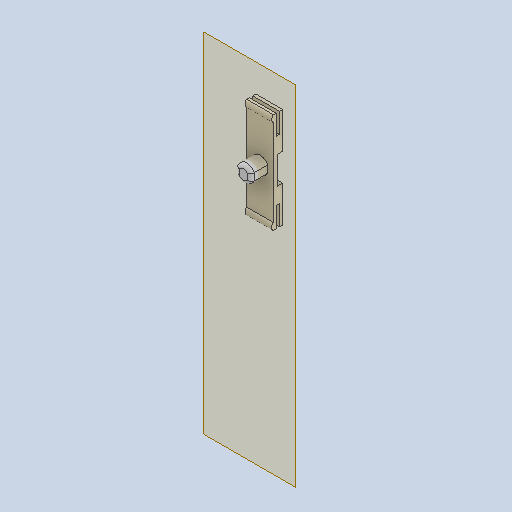
# Autodesk Inventor part: ON_Off_switch
Saved by Autodesk Inventor 2022 (Build 260153000, 153)
## iProperties
Created: 2020-11-26
Part Number: ON_Off_switch
Material: Generic
Document SubType Name: Modeling
Designer: simen
Density: 1 g/cm^3
Appearance: Default
Author: simen
## iProperties of the stored document ON_Off_switch_3DPrint.ipt
Created: 2021-12-08
Part Number: ON_Off_switch_3DPrint
Material: Generic
Document SubType Name: Modeling
Designer: simen
Density: 1 g/cm^3
Appearance: Default
Author: simen
Autodesk Inventor part; units mm, degrees
ref_plane "YZ Plane" through (0, 0, 0) normal (1, 0, 0) x (0, 1, 0)
ref_plane "XZ Plane" through (0, 0, 0) normal (0, 1, 0) x (-1, 0, 0)
ref_plane "XY Plane" through (0, 0, 0) normal (0, 0, 1) x (1, 0, 0)
ref_plane "Work Plane1" through (0, 0, 0) normal (0, 0, 1) x (1, 0, 0)
sketch "Sketch1" plane through (0, 0, 0) normal (0, 0, 1) x (1, 0, 0)
  circle A0 centre (12.6053, 80.6735) radius 2.5
  point P0 (0, 0)
  dimension "d0" = 5
  constraints: 1 centre point
  measures "d0" diameter of A0
extrude "Extrusion1" add sketch "Sketch1" along normal blind 2 and the other way blind 3
sketch "Sketch2" plane through (12.6053, 80.6735, -3) normal (0, 0, -1) x (-1, 0, 0)
  line L0 (-4, -15) -> (4, -15)
  line L1 (4, -15) -> (4, 15)
  line L2 (4, 15) -> (-4, 15)
  line L3 (-4, 15) -> (-4, -15)
  line L4 (-4, -15) -> (4, 15)
  line L5 (-4, -15) -> (27.0483, -15) construction
  circle A0 centre (0, 0) radius 2.5 projected
  point P0 (12.6053, -80.6735)
  dimension "d5" = 8
  dimension "d6" = 30
  constraints: 12 end point, 2 horizontal, 2 parallel, 1 coincident, 1 equal length, 1 midpoint, 1 perpendicular
  measures "d5" distance of L0.start L0.end
  measures "d6" distance of L0.end L1.end
extrude "Extrusion2" add sketch "Sketch2" along normal blind 2.75
sketch "Sketch5" plane through (12.6053, 80.6735, 2) normal (0, 0, 1) x (1, 0, 0)
  line L0 (4, 15) -> (4, -15) projected
  line L1 (-4, -15) -> (-4, 15) projected
  circle A0 centre (0, 0) radius 2.5 projected
  line L2 (-2.25, 1.0897) -> (-2.25, -1.0897)
  line L3 (2.25, 1.0897) -> (2.25, -1.0897)
  circle A1 centre (0, 0) radius 2.5 projected
  point P0 (-12.6053, -80.6735)
  point P1 (2.25, 1.0897)
  point P2 (2.25, -1.0897)
  point P3 (-2.25, -1.0897)
  point P4 (-2.25, 1.0897)
  dimension "d21" = 1.75
  dimension "d22" = 1.75
  constraints: 4 end point, 4 point on circle, 2 parallel, 1 vertical
  measures "d21" distance between parallel lines of L1 L2
  measures "d22" distance between parallel lines of L0 L3
extrude "Extrusion5" cut sketch "Sketch5" against normal up to surface (5 mm away) contours A0 L3 | L2 A0
fillet "Fillet1" radius 1 4 edges at (12.6053, 83.1735, 2) (12.6053, 78.1735, 2) (10.3553, 80.6735, 2) (14.8553, 80.6735, 2)
sketch "Sketch7" plane through (16.6053, 65.6735, -3) normal (1, 0, 0) x (0, 0, -1)
  line L0 (3.95, 19.8) -> (5.45, 19.8) construction
  line L1 (1.25, 19.15) -> (1.25, 10.85)
  line L2 (0, 30) -> (2.75, 30) projected
  line L3 (0, 30) -> (0, 0) projected
  line L4 (0, 0) -> (2.75, 0) projected
  line L5 (2.75, 30) -> (2.75, 0) projected
  line L6 (0, 30) -> (2.75, 30) projected
  line L7 (1.25, 19.15) -> (2.75, 19.15)
  line L8 (2.75, 30) -> (2.75, 0) projected
  line L9 (1.25, 10.85) -> (2.75, 10.85)
  point P0 (-3, -65.6735)
  point P1 (2.75, 10.85)
  point P2 (2.75, 19.15)
  dimension "d31" = 8.3
  dimension "d52" = 1.5
  dimension "d53" = 10.85
  constraints: 8 end point, 2 parallel, 2 point on line, 1 horizontal, 1 perpendicular
  measures "d31" distance of L1.start L1.end
  measures "d52" distance of L1.end L9.end
  measures "d53" distance between parallel lines of L2 L7
extrude "Extrusion7" cut sketch "Sketch7" against normal blind 5 contours L7 L5 L9 L1
chamfer "Chamfer1" distance 0.7 angle 45 1 edges at (11.6053, 80.6735, -4.25)
sketch "Sketch8" plane through (16.6053, 65.6735, -3) normal (1, 0, 0) x (0, 0, -1)
  line L0 (0, 30) -> (2.75, 30) projected
  line L1 (0, 30) -> (0, 0) projected
  line L2 (0, 0) -> (2.75, 0) projected
  line L3 (0, 0) -> (2.75, 0) projected
  line L4 (0, 30) -> (2.75, 30) projected
  line L5 (0.8, 0) -> (0.8, 30)
  line L6 (0, 30) -> (0, 0) projected
  line L7 (1.8, 0) -> (1.8, 30)
  line L8 (0.8, 6) -> (1.8, 6)
  line L9 (0.8, 24) -> (1.8, 24)
  line L10 (2.75, 30) -> (2.75, 19.15) projected
  line L11 (2.75, 10.85) -> (1.25, 10.85) projected
  line L12 (1.25, 10.85) -> (1.25, 19.15) projected
  line L13 (1.25, 19.15) -> (2.75, 19.15) projected
  line L14 (2.75, 10.85) -> (2.75, 0) projected
  point P0 (-3, -65.6735)
  dimension "d38" = 0.8
  dimension "d39" = 1
  dimension "d40" = 6
  dimension "d41" = 6
  dimension "d55" = 0.95
  constraints: 8 end point, 8 point on line, 2 parallel, 2 perpendicular
  measures "d38" distance between parallel lines of L1 L5
  measures "d39" distance between parallel lines of L5 L7
  measures "d40" distance between parallel lines of L2 L8
  measures "d41" distance between parallel lines of L0 L9
  measures "d55" distance between parallel lines of L14 L7
extrude "Extrusion8" cut sketch "Sketch8" against normal up to surface (8 mm away) contours L0 L7 L9 L5 | L5 L8 L7 L2
sketch "Sketch9" plane through (16.6053, 65.6735, -3) normal (1, 0, 0) x (0, 0, -1)
  line L0 (0, 0) -> (0, 30) projected
  line L1 (0, 30) -> (0, 0) projected
  ellipse E0 centre (0, 1) end of major axis (0, 2) minor radius 0.5 (0, 2) -> (0, 0) ccw
  ellipse E1 centre (0, 29) end of major axis (0, 30) minor radius 0.5
  point P0 (-3, -65.6735)
  point P1 (0, 28)
  dimension "d48" = 0.5
  dimension "d49" = 0.5
  dimension "d50" = 1
  dimension "d51" = 1
  constraints: 3 end point, 2 point on line, 2 vertical, 7 other
extrude "Extrusion9" add sketch "Sketch9" against normal up to surface (8 mm away) contours E0 L0 | E1 L0 picked at (-0.1666, 28.9882)
body "Solid1"
